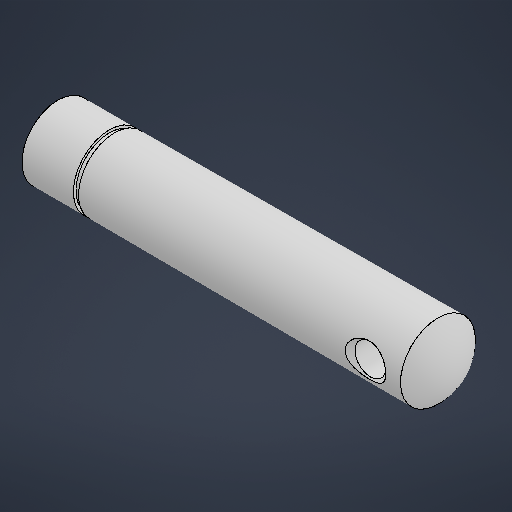
# Autodesk Inventor part: TW1-004B
Saved by Autodesk Inventor 2025.3 (Build 293356000, 356)
## iProperties
Created: 2025-09-14
Part Number: TW1-004B
Material: Generic
Document SubType Name: Modeling
Designer: fablabadmin
Density: 1 g/cm^3
Appearance: Default
Description: Handle type B
Stock Number: C45E
Author: Benjamin Solar
Title: WEDU
Revision Number: 1
Autodesk Inventor part; units mm, degrees
ref_plane "YZ Plane" through (0, 0, 0) normal (1, 0, 0) x (0, 1, 0)
ref_plane "XZ Plane" through (0, 0, 0) normal (0, 1, 0) x (-1, 0, 0)
ref_plane "XY Plane" through (0, 0, 0) normal (0, 0, 1) x (1, 0, 0)
sketch "Sketch1" plane through (0, 0, 0) normal (0, 0, 1) x (1, 0, 0)
  line L0 (-15.5502, 0) -> (93.3013, 0) projected
  line L1 (0, -5.1197) -> (0, 9.718) construction
  line L2 (0, 5.1) -> (0, 7)
  line L3 (0, 7) -> (11, 7)
  line L4 (11, 7) -> (11, 7)
  line L5 (11, 7) -> (73.8618, 7.2743)
  line L6 (73.8618, 7.2743) -> (73.8618, 0) construction
  line L7 (0, 5.1) -> (47.0555, 5.1)
  line L8 (47.0555, 5.1) -> (50, 0)
  arc A0 (77, 0) -> (73.8618, 7.2743) centre (67, 0) ccw
  circle A1 centre (67, 0) radius 3
  line L9 (10, 7) -> (10, 6.5)
  line L10 (10, 6.5) -> (11, 6.5)
  line L11 (11, 6.5) -> (11, 7)
  point P0 (0, 0)
  dimension "d4" = 0.25
  dimension "d5" = 10.2
  dimension "d6" = 14
  dimension "d7" = 14
  dimension "d11" = 50
  dimension "d13" = 60
  dimension "d19" = 10
  dimension "d20" = 77
  dimension "d21" = 67
  dimension "d22" = 6
  dimension "d23" = 0.5
  dimension "d24" = 10
  dimension "d25" = 1
  constraints: 20 end point, 8 point on line, 4 perpendicular, 2 centre point, 2 horizontal, 2 point on circle, 1 vertical
  measures "d4" angle of L0 L5
  measures "d5" diameter of L7 L0
  measures "d6" diameter of L3 L0
  measures "d7" diameter of L4.end L0
  measures "d11" distance from line of L1 L8.end
  measures "d13" angle of L0 L8
  measures "d19" radius of A0
  measures "d20" distance from line of A0.start L1
  measures "d21" distance from line of L1 A1.centre
  measures "d22" diameter of A1
  measures "d23" distance between parallel lines of L3 L10
  measures "d24" distance from line of L1 L9.end
  measures "d25" distance of L9.end L10.end
revolve "Revolution1" add sketch "Sketch1" angle 360 about axis through (-10, 0, 0) along (1, 0, 0) picked at (67.8855, 0.4647) contours A1 L0 L8 L7 L2 L3 L9 L10 L11 L5 A0 | L0 A1
extrude "Extrusion1" cut sketch "Sketch1" along normal through all both and the other way through all contours A1 L0 | L0 A1
sketch "Sketch2" plane through (0, 0, 0) normal (0, 1, 0) x (-1, 0, 0)
  line L0 (-70, -7.2574) -> (-70, 7.2574) projected
  line L1 (-64, -7.2313) -> (-64, 7.2313) projected
  line L2 (-11, 7) -> (-73.8618, 7.2743) projected
  line L3 (-71, 7.2618) -> (-70, 6.253)
  line L4 (-67, 7.2443) -> (-67, -7.2443)
  line L5 (-11, -7) -> (-73.8618, -7.2743) projected
  line L6 (-64, 7.2313) -> (-70, 7.2574)
  point P0 (0, 0)
  dimension "d29" = 45
  dimension "d30" = 1
  constraints: 6 end point, 4 point on line, 1 collinear, 1 midpoint, 1 vertical
  measures "d29" angle of L2 L3
  measures "d30" distance from line of L0 L3.start
revolve "Revolution2" cut sketch "Sketch2" angle 360 about axis through (67, 0, 7.2443) along (0, 0, -1) contours L3 L2 L0
mirror "Mirror1" about plane through (0, 0, 0) normal (0, 0, 1) of "Revolution2"
body "Solid1"
